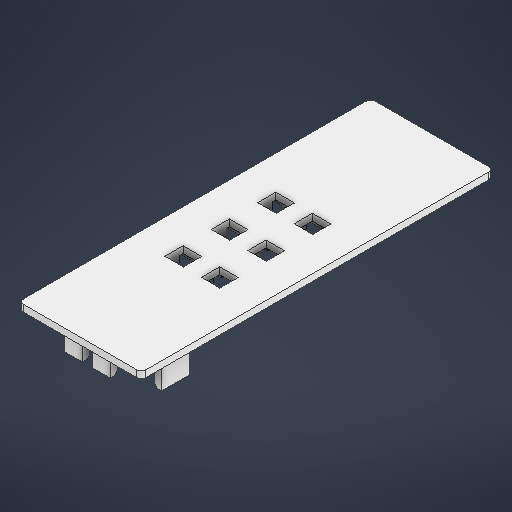
# Autodesk Inventor part: module-lid_switch
Saved by Autodesk Inventor 2025.2 (Build 292293000, 293)
## iProperties
Created: 2025-09-07
Part Number: module-lid_switch
Material: PC/ABS Plastic
Document SubType Name: Modeling
Designer: sam
Density: 1.1 g/cm^3
Appearance: Smooth - White
Author: sam
Autodesk Inventor part; units mm, degrees
ref_plane "YZ Plane" through (0, 0, 0) normal (1, 0, 0) x (0, 1, 0)
ref_plane "XZ Plane" through (0, 0, 0) normal (0, 1, 0) x (-1, 0, 0)
ref_plane "XY Plane" through (0, 0, 0) normal (0, 0, 1) x (1, 0, 0)
sketch "Sketch1" plane through (0, 0, 0) normal (0, 1, 0) x (-1, 0, 0)
  line L0 (-27.2, -78) -> (27.2, -78)
  line L1 (27.2, -78) -> (27.2, 78)
  line L2 (27.2, 78) -> (-27.2, 78)
  line L3 (-27.2, 78) -> (-27.2, -78)
  line L4 (-27.2, -78) -> (27.2, 78) construction
  line L5 (27.2, -78) -> (-27.2, 78) construction
  point P0 (0, 0)
  dimension "d0" = 54.4
  dimension "d1" = 156
  constraints: 12 end point, 2 midpoint, 2 parallel, 1 horizontal, 1 perpendicular
  measures "d0" distance of L2.end L1.end
  measures "d1" distance between parallel lines of L0 L2
extrude "Extrusion1" add sketch "Sketch1" along normal blind 3
sketch "Sketch2" plane through (0, 0, 0) normal (0, -1, 0) x (1, 0, 0)
  line L0 (24, 74.8) -> (-24, 74.8)
  line L1 (-24, 74.8) -> (-24, -74.8)
  line L2 (-24, -74.8) -> (24, -74.8)
  line L3 (24, -74.8) -> (24, 74.8)
  line L4 (24, 74.8) -> (-24, -74.8) construction
  line L5 (-24, 74.8) -> (24, -74.8) construction
  line L6 (-27.2, -78) -> (-27.2, 78) projected
  line L7 (27.2, -78) -> (-27.2, -78) projected
  point P0 (0, 0)
  dimension "d4" = 3.2
  dimension "d5" = 3.2
  constraints: 12 end point, 2 midpoint, 2 parallel, 1 horizontal, 1 perpendicular
  measures "d4" distance between parallel lines of L6 L1
  measures "d5" distance between parallel lines of L7 L2
extrude "Extrusion2" add sketch "Sketch2" along normal blind 3
fillet "Fillet1" radius 2 8 edges at (27.2, 1.5, 78) (24, -1.5, 74.8) (-24, -1.5, 74.8) (-27.2, 1.5, 78) (24, -1.5, -74.8) (27.2, 1.5, -78) (-27.2, 1.5, -78) (-24, -1.5, -74.8)
fillet "Fillet2" radius 0.5 8 edges at (-23.4142, -3, 74.2142) (-24, -3, 0) (-23.4142, -3, -74.2142) (0, -3, -74.8) (23.4142, -3, -74.2142) (24, -3, 0) (23.4142, -3, 74.2142) (0, -3, 74.8)
sketch "Sketch3" plane through (0, -3, 0) normal (0, -1, 0) x (1, 0, 0)
  line L0 (-22, 74.8) -> (22, 74.8) projected
  line L1 (-10.2, 74.8) -> (-2.14, 74.8)
  line L2 (-2.14, 74.8) -> (-2.14, 71.8)
  line L3 (-2.14, 71.8) -> (-10.2, 71.8)
  line L4 (-10.2, 71.8) -> (-10.2, 74.8)
  line L5 (-27.2, -76) -> (-27.2, 76) projected
  line L6 (2.14, 74.8) -> (10.2, 74.8)
  line L7 (10.2, 74.8) -> (10.2, 71.8)
  line L8 (10.2, 71.8) -> (2.14, 71.8)
  line L9 (2.14, 71.8) -> (2.14, 74.8)
  line L10 (27.2, 76) -> (27.2, -76) projected
  point P0 (0, 0)
  dimension "d10" = 8.06
  dimension "d11" = 3
  dimension "d12" = 17
  dimension "d13" = 8.06
  dimension "d14" = 3
  dimension "d15" = 17
  dimension "d17" = 0
  constraints: 16 end point, 4 parallel, 2 horizontal, 2 perpendicular, 1 point on line
  measures "d10" distance of L2.end L3.end
  measures "d11" distance of L1.end L2.end
  measures "d12" distance between parallel lines of L5 L4
  measures "d13" distance of L7.end L8.end
  measures "d14" distance of L6.end L7.end
  measures "d15" distance between parallel lines of L10 L7
  measures "d17" distance between parallel lines of L0 L6
extrude "Extrusion3" add sketch "Sketch3" along normal blind 9.3 from surface at -3
sketch "Sketch4" plane through (0, -3, 0) normal (0, -1, 0) x (1, 0, 0)
  line L0 (24, 72.8) -> (24, -72.8) projected
  line L1 (24, 64.8) -> (20, 64.8)
  line L2 (20, 64.8) -> (20, 52.7)
  line L3 (20, 52.7) -> (24, 52.7)
  line L4 (24, 52.7) -> (24, 64.8)
  line L5 (-24, -72.8) -> (-24, 72.8) projected
  line L6 (-24, 64.8) -> (-20, 64.8)
  line L7 (-20, 64.8) -> (-20, 52.7)
  line L8 (-20, 52.7) -> (-24, 52.7)
  line L9 (-24, 52.7) -> (-24, 64.8)
  line L10 (-25.2, 78) -> (25.2, 78) projected
  line L11 (-10.2, 74.8) -> (-22, 74.8) projected
  line L12 (22, 74.8) -> (10.2, 74.8) projected
  line L13 (-24, 52.7) -> (-23, 52.7)
  line L14 (-23, 52.7) -> (-23, 64.8)
  line L15 (-23, 64.8) -> (-24, 64.8)
  line L16 (-24, 64.8) -> (-24, 52.7)
  line L17 (24, 52.7) -> (23, 52.7)
  line L18 (23, 52.7) -> (23, 64.8)
  line L19 (23, 64.8) -> (24, 64.8)
  line L20 (24, 64.8) -> (24, 52.7)
  point P0 (0, 0)
  dimension "d23" = 4
  dimension "d24" = 12.1
  dimension "d25" = 4
  dimension "d26" = 12.1
  dimension "d29" = 10
  dimension "d30" = 10
  dimension "d31" = 1
  dimension "d32" = 1
  constraints: 32 end point, 8 parallel, 4 horizontal, 4 perpendicular, 4 point on line
  measures "d23" distance of L3.end L2.end
  measures "d24" distance of L2.end L1.end
  measures "d25" distance of L7.end L8.end
  measures "d26" distance of L6.end L7.end
  measures "d29" distance between parallel lines of L11 L6
  measures "d30" distance between parallel lines of L12 L1
  measures "d31" distance of L15.end L14.end
  measures "d32" distance of L18.end L19.end
extrude "Extrusion4" add sketch "Sketch4" along normal blind 12.8 from surface at -3 contours L18 L3 L2 L1 | L14 L6 L7 L8
chamfer "Chamfer1" distance 1 angle 45 4 edges at (-6.17, -9.3, 71.8) (6.17, -9.3, 71.8) (-20, -12.8, 58.75) (20, -12.8, 58.75)
sketch "Sketch5" plane through (0, 3, 0) normal (0, 1, 0) x (1, 0, 0)
  arc A0 (-25.2, 78) -> (-27.2, 76) centre (-25.2, 76) ccw projected
  line L0 (-27.2, 76) -> (-27.2, -76) projected
  arc A1 (-27.2, -76) -> (-25.2, -78) centre (-25.2, -76) ccw projected
  line L1 (-25.2, -78) -> (25.2, -78) projected
  arc A2 (25.2, -78) -> (27.2, -76) centre (25.2, -76) ccw projected
  line L2 (27.2, -76) -> (27.2, 76) projected
  arc A3 (27.2, 76) -> (25.2, 78) centre (25.2, 76) ccw projected
  line L3 (25.2, 78) -> (-25.2, 78) projected
  line L4 (-12.2, 21) -> (-4, 21)
  line L5 (-4, 21) -> (-4, 12.94)
  line L6 (-4, 12.94) -> (-12.2, 12.94)
  line L7 (-12.2, 12.94) -> (-12.2, 21)
  line L8 (12.2, 21) -> (4, 21)
  line L9 (4, 21) -> (4, 12.94)
  line L10 (4, 12.94) -> (12.2, 12.94)
  line L11 (12.2, 12.94) -> (12.2, 21)
  line L12 (-12.2, 0.44) -> (-4, 0.44)
  line L13 (-4, 0.44) -> (-4, -7.62)
  line L14 (-4, -7.62) -> (-12.2, -7.62)
  line L15 (-12.2, -7.62) -> (-12.2, 0.44)
  line L16 (12.2, 0.44) -> (4, 0.44)
  line L17 (4, 0.44) -> (4, -7.62)
  line L18 (4, -7.62) -> (12.2, -7.62)
  line L19 (12.2, -7.62) -> (12.2, 0.44)
  line L20 (-12.2, -20.12) -> (-4, -20.12)
  line L21 (-4, -20.12) -> (-4, -28.18)
  line L22 (-4, -28.18) -> (-12.2, -28.18)
  line L23 (-12.2, -28.18) -> (-12.2, -20.12)
  line L24 (12.2, -20.12) -> (4, -20.12)
  line L25 (4, -20.12) -> (4, -28.18)
  line L26 (4, -28.18) -> (12.2, -28.18)
  line L27 (12.2, -28.18) -> (12.2, -20.12)
  point P0 (0, 0)
  dimension "d35" = 8.2
  dimension "d36" = 8.06
  dimension "d37" = 57
  dimension "d38" = 15
  dimension "d39" = 8.2
  dimension "d40" = 57
  dimension "d41" = 15
  dimension "d42" = 8.06
  dimension "d45" = 8.2
  dimension "d46" = 8.06
  dimension "d47" = 8.2
  dimension "d48" = 8.06
  dimension "d49" = 8.2
  dimension "d50" = 8.06
  dimension "d51" = 8.2
  dimension "d52" = 8.06
  dimension "d57" = 15
  dimension "d58" = 15
  dimension "d59" = 15
  dimension "d60" = 15
  dimension "d61" = 12.5
  dimension "d62" = 12.5
  dimension "d63" = 12.5
  dimension "d64" = 12.5
  constraints: 48 end point, 12 parallel, 6 horizontal, 6 perpendicular
  measures "d35" distance of L5.end L6.end
  measures "d36" distance of L4.end L5.end
  measures "d37" distance between parallel lines of L3 L4
  measures "d38" distance between parallel lines of L0 L7
  measures "d39" distance of L10.end L9.end
  measures "d40" distance between parallel lines of L3 L8
  measures "d41" distance between parallel lines of L2 L11
  measures "d42" distance between parallel lines of L8 L10
  measures "d45" distance of L14.start L14.end
  measures "d46" distance of L13.start L14.start
  measures "d47" distance of L18.end L18.start
  measures "d48" distance between parallel lines of L16 L18
  measures "d49" distance of L22.start L22.end
  measures "d50" distance of L21.start L22.start
  measures "d51" distance of L26.end L26.start
  measures "d52" distance between parallel lines of L24 L26
  measures "d57" distance between parallel lines of L0 L15
  measures "d58" distance between parallel lines of L2 L19
  measures "d59" distance between parallel lines of L2 L27
  measures "d60" distance between parallel lines of L0 L23
  measures "d61" distance between parallel lines of L6 L12
  measures "d62" distance between parallel lines of L10 L16
  measures "d63" distance between parallel lines of L14 L20
  measures "d64" distance between parallel lines of L18 L24
extrude "Extrusion5" cut sketch "Sketch5" against normal through all contours L4 L5 L6 L7 | L11 L10 L9 L8 | L12 L13 L14 L15 | L19 L18 L17 L16 | L20 L21 L22 L23 | L27 L26 L25 L24
sketch "Sketch6" plane through (0, -3, 0) normal (0, -1, 0) x (1, 0, 0)
  line L0 (8.2, -20.6) -> (2.8, -20.6)
  line L1 (2.8, -20.6) -> (2.8, 29.4)
  line L2 (2.8, 29.4) -> (8.2, 29.4)
  line L3 (8.2, 29.4) -> (8.2, -20.6)
  line L4 (-8.2, 29.4) -> (-2.8, 29.4)
  line L5 (-2.8, 29.4) -> (-2.8, -20.6)
  line L6 (-2.8, -20.6) -> (-8.2, -20.6)
  line L7 (-8.2, -20.6) -> (-8.2, 29.4)
  line L8 (26, -19.6) -> (-26, -19.6)
  line L9 (-26, -19.6) -> (-26, -23)
  line L10 (-26, -23) -> (26, -23)
  line L11 (26, -23) -> (26, -19.6)
  line L12 (2.8, -20.6) -> (-2.8, -20.6)
  line L13 (26, -2.44) -> (-26, -2.44)
  line L14 (-26, -2.44) -> (-26, 0.96)
  line L15 (-26, 0.96) -> (26, 0.96)
  line L16 (26, 0.96) -> (26, -2.44)
  line L17 (26, 18.12) -> (-26, 18.12)
  line L18 (-26, 18.12) -> (-26, 21.52)
  line L19 (-26, 21.52) -> (26, 21.52)
  line L20 (26, 21.52) -> (26, 18.12)
  line L21 (25.2, -78) -> (-25.2, -78) projected
  line L22 (27.2, 76) -> (27.2, -76) projected
  point P0 (0, 0)
  point P1 (0, -20.6)
  point P2 (0, -23)
  point P3 (0, -2.44)
  point P4 (8.2, -2.44)
  point P5 (8.2, 0.96)
  point P6 (8.2, 18.12)
  point P7 (8.2, 21.52)
  point P8 (2.8, 21.52)
  point P9 (-2.8, 21.52)
  point P10 (-8.2, 21.52)
  point P11 (-8.2, 18.12)
  point P12 (-8.2, 0.96)
  point P13 (-8.2, -2.44)
  point P14 (-8.2, -19.6)
  point P15 (8.2, -19.6)
  point P16 (2.8, 0.96)
  point P17 (-2.8, 0.96)
  point P18 (-2.8, 18.12)
  point P19 (2.8, 18.12)
  point P20 (2.8, -2.44)
  point P21 (2.8, -19.6)
  point P22 (-2.8, -19.6)
  point P23 (-2.8, -2.44)
  dimension "d65" = 5.4
  dimension "d66" = 50
  dimension "d67" = 5.4
  dimension "d68" = 50
  dimension "d69" = 52
  dimension "d70" = 3.4
  dimension "d71" = 1
  dimension "d72" = 0
  dimension "d73" = 52
  dimension "d74" = 3.4
  dimension "d75" = 52
  dimension "d76" = 3.4
  dimension "d77" = 20.56
  dimension "d78" = 20.56
  dimension "d79" = 16.4
  dimension "d80" = 0
  dimension "d81" = 55
  dimension "d82" = 1.2
  constraints: 42 end point, 10 parallel, 5 horizontal, 5 perpendicular, 3 midpoint, 1 collinear, 1 point on line
  measures "d65" distance of L1.end L3.start
  measures "d66" distance of L0.end L1.end
  measures "d67" distance between parallel lines of L7 L5
  measures "d68" distance between parallel lines of L4 L6
  measures "d69" distance of L11.start L9.end
  measures "d70" distance of L9.end L9.start
  measures "d71" distance between parallel lines of L6 L8
  measures "d72" horizontal distance of point (0, -20.6) point (0, -23)
  measures "d73" distance of L14.end L16.start
  measures "d74" distance of L14.start L14.end
  measures "d75" distance of L19.start L20.start
  measures "d76" distance of L18.start L19.start
  measures "d77" distance between parallel lines of L15 L8
  measures "d78" distance between parallel lines of L19 L15
  measures "d79" distance between parallel lines of L7 L3
  measures "d80" horizontal distance of point (0, -20.6) point (0, -2.44)
  measures "d81" distance between parallel lines of L21 L10
  measures "d82" distance between parallel lines of L22 L11
extrude "Extrusion6" cut sketch "Sketch6" against normal blind 3 contours L3 L8 L11 L10 L9 L7 L6 L12 L0 | L0 L1 L8 L3 | L12 L5 L8 L1 | L8 L1 L13 L3 | L6 L7 L8 L5 | L13 L1 L15 L3 | L3 L15 L16 L13 | L13 L5 L15 L1 | L8 L7 L13 L5 | L15 L1 L17 L3 | L13 L7 L15 L5 | L17 L1 L19 L3 | L3 L19 L20 L17 | L17 L5 L19 L1 | L15 L7 L17 L5 | L13 L14 L15 L7 | L19 L1 L2 L3 | L17 L7 L19 L5 | L19 L7 L4 L5 | L17 L18 L19 L7
equation "\"d62\" = d61"
equation "\"d63\" = d61"
equation "\"d64\" = d63"
equation "\"d67\" = d65"
equation "\"d68\" = d66"
body "Solid1"
